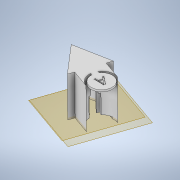
# Autodesk Inventor part: Wire_Closing_4
Saved by Autodesk Inventor 2022.3 (Build 263350000, 350)
## iProperties
Created: 2023-05-15
Part Number: Wire_Closing_4
Material: Generic
Document SubType Name: Modeling
Designer: Manuel Hueso Béjar
Density: 1 g/cm^3
Appearance: Default
Author: Manuel Hueso Béjar
Autodesk Inventor part; units mm, degrees
ref_plane "YZ Plane" through (0, 0, 0) normal (1, 0, 0) x (0, 1, 0)
ref_plane "XZ Plane" through (0, 0, 0) normal (0, 1, 0) x (-1, 0, 0)
ref_plane "XY Plane" through (0, 0, 0) normal (0, 0, 1) x (1, 0, 0)
ref_plane "Work Plane1" through (99.4089, 148.8532, -64.157) normal (-0.0019043, 0.9999705, 0.007443) x (-0.9432702, 0.000675, -0.3320254)
sketch "Sketch1" plane through (99.4089, 148.8532, -64.157) normal (-0.0019043, 0.9999705, 0.007443) x (-0.9432702, 0.000675, -0.3320254)
  arc A0 (-20.1728, 11.5) -> (-26.235, 13) centre (-26.235, 0) ccw projected
  line L0 (-5.235, 11.5) -> (-20.1728, 11.5) projected
  line L1 (-5.235, 16.4372) -> (-5.235, 11.5) projected
  line L2 (23.235, 0) -> (-5.235, 16.4372) projected
  line L3 (-5.235, -16.4372) -> (23.235, 0) projected
  line L4 (-5.235, -11.5) -> (-5.235, -16.4372) projected
  line L5 (-20.1728, -11.5) -> (-5.235, -11.5) projected
  arc A1 (-26.235, -13) -> (-20.1728, -11.5) centre (-26.235, 0) ccw projected
  line L6 (-6.735, -13) -> (-26.235, -13) projected
  line L7 (-6.735, -19.0353) -> (-6.735, -13) projected
  line L8 (26.235, 0) -> (-6.735, -19.0353) projected
  line L9 (-6.735, 19.0353) -> (26.235, 0) projected
  line L10 (-6.735, 13) -> (-6.735, 19.0353) projected
  line L11 (-26.235, 13) -> (-6.735, 13) projected
  point P0 (72.3673, 94.6605)
extrude "Extrusion1" add sketch "Sketch1" along normal blind 42
ref_plane "Work Plane2" through (105.5364, 150.8487, -61.984) normal (-0.0019043, 0.9999705, 0.007443) x (-0.9432702, 0.000675, -0.3320254)
sketch "Sketch2" plane through (105.5364, 150.8487, -61.984) normal (-0.0019043, 0.9999705, 0.007443) x (-0.9432702, 0.000675, -0.3320254)
  circle A0 centre (-19.735, 0) radius 4.1 projected
  line L0 (-13.6728, -11.5) -> (1.265, -11.5) projected
  line L1 (1.265, -11.5) -> (1.265, -16.4372) projected
  line L2 (1.265, -16.4372) -> (29.735, 0) projected
  line L3 (29.735, 0) -> (1.265, 16.4372) projected
  line L4 (1.265, 16.4372) -> (1.265, 11.5) projected
  line L5 (1.265, 11.5) -> (-13.6728, 11.5) projected
  arc A1 (-7.735, 5) -> (-13.6728, 11.5) centre (-19.735, 0) ccw projected
  line L6 (-7.735, 5) -> (-6.0859, 5) projected
  line L7 (-6.0859, 5) -> (-4.0859, 7) projected
  line L8 (-4.0859, 7) -> (-4.0859, 3) projected
  line L9 (-4.0859, 3) -> (-9.152, 3) projected
  arc A2 (-9.152, 3) -> (-9.152, -3) centre (-19.735, 0) ccw projected
  line L10 (-9.152, -3) -> (-4.0859, -3) projected
  line L11 (-4.0859, -3) -> (-4.0859, -7) projected
  line L12 (-4.0859, -7) -> (-6.0859, -5) projected
  line L13 (-6.0859, -5) -> (-7.735, -5) projected
  arc A3 (-13.6728, -11.5) -> (-7.735, -5) centre (-19.735, 0) ccw projected
  circle A4 centre (4.765, 0) radius 7 projected
  line L14 (-6.5001, -6) -> (-3.0859, -9.4142)
  line L15 (-3.0859, -9.4142) -> (-3.0859, -2)
  line L16 (-3.0859, -2) -> (-9.9371, -2)
  arc A5 (-9.9371, 2) -> (-9.9371, -2) centre (-19.735, 0) ccw
  line L17 (-9.9371, 2) -> (-3.0859, 2)
  line L18 (-3.0859, 2) -> (-3.0859, 9.4142)
  line L19 (-3.0859, 9.4142) -> (-6.5001, 6)
  line L20 (-6.5001, 6) -> (-7.0859, 6)
  arc A6 (-7.0859, 6) -> (-10.4749, 10.5) centre (-19.735, 0) ccw
  line L21 (-10.4749, 10.5) -> (2.265, 10.5)
  line L22 (2.265, 10.5) -> (2.265, 14.7051)
  line L23 (2.265, 14.7051) -> (27.735, 0)
  line L24 (27.735, 0) -> (2.265, -14.7051)
  line L25 (2.265, -14.7051) -> (2.265, -10.5)
  line L26 (2.265, -10.5) -> (-10.4749, -10.5)
  arc A7 (-10.4749, -10.5) -> (-7.0859, -6) centre (-19.735, 0) ccw
  line L27 (-7.0859, -6) -> (-6.5001, -6)
  line L28 (-3.0859, -9.4142) -> (-3.0859, -11.5)
  line L29 (1.265, -11.5) -> (-13.6728, -11.5) projected
  line L30 (-4.0859, -3) -> (-3.0859, -3)
  line L31 (-3.0859, 9.4142) -> (-3.0859, 11.5)
  line L32 (-13.6728, 11.5) -> (1.265, 11.5) projected
  line L33 (-4.0859, 3) -> (-3.0859, 3)
  point P0 (78.8673, 94.6605)
  point P1 (-3.0859, 11.5)
  point P2 (-3.0859, -11.5)
  dimension "d2" = 1
  constraints: 36 end point, 6 point on circle, 5 point on line, 3 centre point, 3 perpendicular, 16 other
  measures "d2" distance between parallel lines of L12 L14
extrude "Extrusion2" add sketch "Sketch2" along normal blind 20 contours A3 L13 L12 L11 L30 L15 L14 L27 A7 L26 L28 L0 | L26 A7 L27 L14 L28 | L31 L21 A6 L20 L19 L18 L33 L8 L7 L6 A1 L5 | L31 L19 L20 A6 L21
sketch "Sketch3" plane through (105.4983, 170.8481, -61.8351) normal (-0.0019043, 0.9999705, 0.007443) x (0.9432702, -0.000675, 0.3320254)
  line L0 (4.0859, 7) -> (6.0859, 5) projected
  line L1 (6.0859, 5) -> (7.735, 5) projected
  arc A0 (13.6728, 11.5) -> (7.735, 5) centre (19.735, 0) ccw projected
  line L2 (3.0859, 11.5) -> (13.6728, 11.5) projected
  line L3 (3.0859, 11.5) -> (3.0859, 3) projected
  line L4 (3.0859, 3) -> (4.0859, 3) projected
  line L5 (4.0859, 3) -> (4.0859, 7) projected
  circle A1 centre (19.735, 0) radius 4.1 projected
  line L6 (13.6728, 11.5) -> (-1.265, 11.5) projected
  line L7 (-1.265, 11.5) -> (-1.265, 16.4372) projected
  line L8 (-1.265, 16.4372) -> (-29.735, 0) projected
  line L9 (-29.735, 0) -> (-1.265, -16.4372) projected
  line L10 (-1.265, -16.4372) -> (-1.265, -11.5) projected
  line L11 (-1.265, -11.5) -> (13.6728, -11.5) projected
  arc A2 (7.735, -5) -> (13.6728, -11.5) centre (19.735, 0) ccw projected
  line L12 (7.735, -5) -> (6.0859, -5) projected
  line L13 (6.0859, -5) -> (4.0859, -7) projected
  line L14 (4.0859, -7) -> (4.0859, -3) projected
  line L15 (4.0859, -3) -> (9.152, -3) projected
  arc A3 (9.152, -3) -> (9.152, 3) centre (19.735, 0) ccw projected
  line L16 (9.152, 3) -> (4.0859, 3) projected
  line L17 (4.0859, 3) -> (4.0859, 7) projected
  line L18 (4.0859, 7) -> (6.0859, 5) projected
  line L19 (6.0859, 5) -> (7.735, 5) projected
  arc A4 (13.6728, 11.5) -> (7.735, 5) centre (19.735, 0) ccw projected
  circle A5 centre (-4.765, 0) radius 7 projected
  line L20 (7.735, 5) -> (7.735, 3)
  line L21 (7.735, -5) -> (6.0859, -5) projected
  line L22 (7.735, -5) -> (7.735, -3)
  line L23 (7.735, -5) -> (6.0859, -5) projected
  line L24 (6.0859, -5) -> (4.0859, -7) projected
  line L25 (4.0859, -7) -> (4.0859, -3) projected
  line L26 (4.0859, -3) -> (3.0859, -3) projected
  line L27 (3.0859, -3) -> (3.0859, -11.5) projected
  line L28 (13.6728, -11.5) -> (3.0859, -11.5) projected
  arc A6 (7.735, -5) -> (13.6728, -11.5) centre (19.735, 0) ccw projected
  arc A7 (9.152, -3) -> (9.152, 3) centre (19.735, 0) ccw projected
  line L29 (9.152, -3) -> (7.0859, -3) projected
  arc A8 (7.0859, -3) -> (7.0859, 3) centre (19.735, 0) ccw projected
  line L30 (7.0859, 3) -> (9.152, 3) projected
  point P0 (-78.8673, -94.6605)
  point P1 (4.0859, -3)
  point P2 (3.0859, -11.5)
  constraints: 4 end point, 2 perpendicular, 2 point on line
extrude "Extrusion3" add sketch "Sketch3" along normal up to surface (20 mm away) contours L5 L4 L3 L2 A0 L1 L0 | L0 L1 A8 L16 L5 | L11 L27 L26 L14 L13 L12 A2 | L12 L13 L14 L15 A8
sketch "Sketch4" plane through (99.329, 190.8519, -63.8444) normal (-0.0019043, 0.9999705, 0.007443) x (0.9432702, -0.000675, 0.3320254)
  circle A0 centre (26.235, 0) radius 4.1 projected
  line L0 (20.1728, 11.5) -> (5.235, 11.5) projected
  line L1 (5.235, 11.5) -> (5.235, 16.4372) projected
  line L2 (5.235, 16.4372) -> (-23.235, 0) projected
  line L3 (-23.235, 0) -> (5.235, -16.4372) projected
  line L4 (5.235, -16.4372) -> (5.235, -11.5) projected
  line L5 (5.235, -11.5) -> (20.1728, -11.5) projected
  arc A1 (14.235, -5) -> (20.1728, -11.5) centre (26.235, 0) ccw projected
  line L6 (14.235, -5) -> (12.5859, -5) projected
  line L7 (12.5859, -5) -> (10.5859, -7) projected
  line L8 (10.5859, -7) -> (10.5859, -3) projected
  line L9 (10.5859, -3) -> (15.652, -3) projected
  arc A2 (15.652, -3) -> (15.652, 3) centre (26.235, 0) ccw projected
  line L10 (15.652, 3) -> (10.5859, 3) projected
  line L11 (10.5859, 3) -> (10.5859, 7) projected
  line L12 (10.5859, 7) -> (12.5859, 5) projected
  line L13 (12.5859, 5) -> (14.235, 5) projected
  arc A3 (20.1728, 11.5) -> (14.235, 5) centre (26.235, 0) ccw projected
  circle A4 centre (1.735, 0) radius 7 projected
  arc A5 (15.652, -3) -> (15.652, 3) centre (26.235, 0) ccw projected
  line L14 (15.652, -3) -> (13.5859, -3) projected
  arc A6 (13.5859, -3) -> (13.5859, 3) centre (26.235, 0) ccw projected
  line L15 (13.5859, 3) -> (15.652, 3) projected
  point P0 (-72.3673, -94.6605)
extrude "Extrusion4" add sketch "Sketch4" against normal blind 2 contours A0 | A3 L13 L12 L11 L10 A2 L9 L8 L7 L6 A1 L5 L4 L3 L2 L1 L0 | A6 L10 L11 L12 L13 | L6 L7 L8 L9 A6 | A4
sketch "Sketch5" plane through (99.329, 190.8519, -63.8444) normal (-0.0019043, 0.9999705, 0.007443) x (0.9432702, -0.000675, 0.3320254)
  line L0 (37.235, 11) -> (37.235, -11) construction
  line L1 (37.235, -11) -> (15.235, -11) construction
  line L2 (15.235, -11) -> (15.235, 11) construction
  line L3 (15.235, 11) -> (37.235, 11) construction
  line L4 (15.235, 11) -> (37.235, 11)
  line L5 (37.235, 11) -> (37.235, -11)
  line L6 (37.235, -11) -> (15.235, -11)
  line L7 (15.235, -11) -> (15.235, 11)
  arc A0 (15.652, -3) -> (15.652, 3) centre (26.235, 0) ccw projected
  line L8 (15.235, 11) -> (37.235, -11) construction
  line L9 (37.235, 11) -> (15.235, -11) construction
  line L10 (21.235, 4.2545) -> (31.235, 0.8833)
  line L11 (31.235, 0.8833) -> (31.235, -0.7536)
  line L12 (31.235, -0.7536) -> (21.235, -4.1248)
  line L13 (21.235, -4.1248) -> (21.235, -2.7229)
  line L14 (21.235, -2.7229) -> (24.0308, -1.8152)
  line L15 (24.0308, -1.8152) -> (24.0308, 2.0016)
  line L16 (24.0308, 2.0016) -> (21.235, 2.9092)
  line L17 (21.235, 2.9092) -> (21.235, 4.2545)
  line L18 (25.1653, -1.4506) -> (29.8736, 0.0972)
  line L19 (29.8736, 0.0972) -> (25.1653, 1.637)
  line L20 (25.1653, 1.637) -> (25.1653, -1.4506)
  point P0 (-72.3673, -94.6605)
  dimension "d9" = 22
  dimension "d10" = 22
  dimension "d11" = 22
  dimension "d12" = 22
  dimension "d13" = 0
  dimension "d14" = 0
  constraints: 12 end point, 2 midpoint, 2 parallel, 1 horizontal, 1 perpendicular, 2 other
  measures "d9" distance of L5.end L6.end
  measures "d10" distance of L4.end L5.end
  measures "d11" distance of L0.start L0.end
  measures "d12" distance of L0.end L1.end
  measures "d13" distance between parallel lines of L5 L0
  measures "d14" distance between parallel lines of L4 L3
emboss "Emboss1" sketch "Sketch5" operation cut depth 1 direction (0.0019043, -0.9999705, -0.007443) contours L10 L11 L12 L13 L14 L15 L16 L17
body "Solid1"
